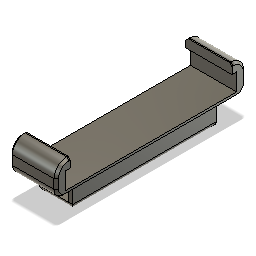
phonemount (Autodesk Fusion 360 design; units mm, degrees)
Autodesk Fusion 360 part; units mm, degrees
sketch "Sketch1" plane through (0, 0, 0) normal (0, 1, 0) x (1, 0, 0)
  line L0 (-28.2713, 23.2028) -> (-13.7713, 23.2028)
  line L1 (-13.7713, 23.2028) -> (-13.7713, -39.2972)
  line L2 (-13.7713, -39.2972) -> (-28.2713, -39.2972)
  line L3 (-28.2713, -39.2972) -> (-28.2713, 23.2028)
  dimension "d1" = 14.5
  dimension "d2" = 62.5
  constraint horizontal L0
  constraint vertical L1
  constraint horizontal L2
  constraint vertical L3
  measures "d1" distance of L0.start L0.end
  measures "d2" distance of L0.start L2.end
extrude "Extrude1" add sketch "Sketch1" along normal blind 9.5
sketch "Sketch3" plane through (0, 0, 39.2972) normal (0, 0, 1) x (1, 0, 0)
  line L0 (-28.2713, 0) -> (-13.7713, 0)
  line L1 (-13.7713, 0) -> (-13.7713, 9.5)
  line L2 (-13.7713, 9.5) -> (-28.2713, 9.5)
  line L3 (-28.2713, 9.5) -> (-28.2713, 0)
  line L4 (-26.2713, 7.5) -> (-15.7713, 7.5)
  line L5 (-15.7713, 7.5) -> (-15.7713, 2)
  line L6 (-15.7713, 2) -> (-26.2713, 2)
  line L7 (-26.2713, 2) -> (-26.2713, 7.5)
  line L8 (-26.2713, 7.5) -> (-15.7713, 2)
  line L9 (-28.2713, 0) -> (-13.7713, 9.5)
  dimension "d7" = 10.5
  dimension "d8" = 5.5
  constraint horizontal L4
  constraint vertical L5
  constraint horizontal L6
  constraint vertical L7
  constraint coincident L0.start L3.end
  constraint coincident L1.end L2.start
  constraint midpoint L8 L9
  measures "d7" distance of L4.start L4.end
  measures "d8" distance of L4.start L6.end
extrude "Extrude2" cut sketch "Sketch3" against normal up to surface (62.5 mm away) contours L6 L8 L9 | L6 L7 L8 L9 | L4 L5 L8 L9 | L4 L8 L9
sketch "Sketch4" plane through (0, 9.5, 0) normal (0, 1, 0) x (-1, 0, 0)
  line L0 (28.2713, 39.2972) -> (13.7713, 39.2972)
  line L1 (13.7713, 39.2972) -> (13.7713, -23.2028)
  line L2 (13.7713, -23.2028) -> (28.2713, -23.2028)
  line L3 (28.2713, -23.2028) -> (28.2713, 39.2972)
  line L4 (31.0213, -33.0528) -> (11.0213, -33.0528)
  line L5 (11.0213, -33.0528) -> (11.0213, 49.1472)
  line L6 (11.0213, 49.1472) -> (31.0213, 49.1472)
  line L7 (31.0213, 49.1472) -> (31.0213, -33.0528)
  line L8 (28.2713, -23.2028) -> (13.7713, 39.2972)
  line L9 (11.0213, -33.0528) -> (31.0213, 49.1472)
  dimension "d11" = 20
  dimension "d12" = 82.2
  constraint horizontal L4
  constraint vertical L5
  constraint horizontal L6
  constraint vertical L7
  constraint coincident L2.end L3.start
  constraint coincident L0.end L1.start
  constraint midpoint L8 L9
  measures "d11" distance of L4.start L4.end
  measures "d12" distance of L4.start L6.end
extrude "Extrude3" add sketch "Sketch4" along normal blind 2
sketch "Sketch8" plane through (0, 11.5, 0) normal (0, 1, 0) x (-1, 0, 0)
  line L0 (31.0213, 49.1472) -> (11.0213, 49.1472)
  line L1 (11.0213, 49.1472) -> (11.0213, -33.0528)
  line L2 (11.0213, -33.0528) -> (31.0213, -33.0528)
  line L3 (31.0213, -33.0528) -> (31.0213, 49.1472)
  line L4 (31.0213, -33.0528) -> (11.0213, -33.0528)
  line L5 (11.0213, -33.0528) -> (11.0213, -29.0528)
  line L6 (11.0213, -29.0528) -> (31.0213, -29.0528)
  line L7 (31.0213, -29.0528) -> (31.0213, -33.0528)
  line L8 (11.0213, 49.1472) -> (31.0213, 49.1472)
  line L9 (31.0213, 49.1472) -> (31.0213, 45.1472)
  line L10 (31.0213, 45.1472) -> (11.0213, 45.1472)
  line L11 (11.0213, 45.1472) -> (11.0213, 49.1472)
  dimension "d26" = 4
  dimension "d27" = 4
  constraint horizontal L4
  constraint vertical L5
  constraint horizontal L6
  constraint vertical L7
  constraint coincident L2.end L3.start
  constraint horizontal L8
  constraint vertical L9
  constraint horizontal L10
  constraint vertical L11
  constraint coincident L0.end L1.start
  measures "d26" distance of L2.end L6.end
  measures "d27" distance of L0.end L10.end
extrude "Extrude7" add sketch "Sketch8" along normal blind 11.5 contours L0 L1 L3 L8 L9 L10 L11 | L1 L2 L3 L4 L5 L6 L7
sketch "Sketch9" plane through (0, 0, -29.0528) normal (0, 0, 1) x (1, 0, 0)
  line L0 (-31.0213, 11.5) -> (-11.0213, 11.5)
  line L1 (-11.0213, 11.5) -> (-11.0213, 23)
  line L2 (-11.0213, 23) -> (-31.0213, 23)
  line L3 (-31.0213, 23) -> (-31.0213, 11.5)
  line L4 (-31.0213, 23) -> (-11.0213, 23)
  line L5 (-11.0213, 23) -> (-11.0213, 19)
  line L6 (-11.0213, 19) -> (-31.0213, 19)
  line L7 (-31.0213, 19) -> (-31.0213, 23)
  dimension "d30" = 4
  constraint horizontal L4
  constraint vertical L5
  constraint horizontal L6
  constraint vertical L7
  constraint coincident L2.end L3.start
  measures "d30" distance of L2.end L6.end
sketch "Sketch10" plane through (0, 0, 45.1472) normal (0, 0, -1) x (-1, 0, 0)
  line L0 (11.0213, 11.5) -> (31.0213, 11.5)
  line L1 (31.0213, 11.5) -> (31.0213, 23)
  line L2 (31.0213, 23) -> (11.0213, 23)
  line L3 (11.0213, 23) -> (11.0213, 11.5)
  line L4 (11.0213, 23) -> (31.0213, 23)
  line L5 (31.0213, 23) -> (31.0213, 19)
  line L6 (31.0213, 19) -> (11.0213, 19)
  line L7 (11.0213, 19) -> (11.0213, 23)
  dimension "d31" = 4
  constraint horizontal L4
  constraint vertical L5
  constraint horizontal L6
  constraint vertical L7
  constraint coincident L2.end L3.start
  measures "d31" distance of L2.end L6.end
extrude "Extrude8" add sketch "Sketch9" along normal blind 2 contours L1 L2 L3 L4 L5 L6 L7
extrude "Extrude9" add sketch "Sketch10" along normal blind 2 contours L1 L2 L3 L4 L5 L6 L7
fillet "Fillet1" radius 2 4 edges at (-13.7713, 0, 8.0472) (-28.2713, 0, 8.0472) (-21.0213, 0, 39.2972) (-21.0213, 0, -23.2028)
fillet "Fillet2" radius 5.5 2 edges at (-21.0213, 23, 49.1472) (-21.0213, 23, -33.0528)
fillet "Fillet3" radius 4 2 edges at (-21.0213, 9.5, -33.0528) (-21.0213, 9.5, 49.1472)
chamfer "Chamfer1" distance 1 angle 45 18 edges at (-31.0213, 23, 43.3972) (-31.0213, 21.3891, 47.5363) (-31.0213, 15.5, 49.1472) (-31.0213, 10.6716, 47.9756) (-31.0213, 9.5, 8.0472) (-31.0213, 10.6716, -31.8812) (-31.0213, 15.5, -33.0528) (-31.0213, 21.3891, -31.4419) (-31.0213, 23, -27.3028) (-11.0213, 23, -27.3028) (-11.0213, 21.3891, -31.4419) (-11.0213, 15.5, -33.0528) (-11.0213, 10.6716, -31.8812) (-11.0213, 9.5, 8.0472) (-11.0213, 10.6716, 47.9756) (-11.0213, 15.5, 49.1472) (-11.0213, 21.3891, 47.5363) (-11.0213, 23, 43.3972)
equation "d1 = 10.5 mm + 4 mm"
equation "d3 = 2 mm + 5.5 mm + 2 mm"
equation "d12 = 73.9 mm + 8 mm + 0.3 mm"
equation "d28 = 7.5 mm + 4 mm"
